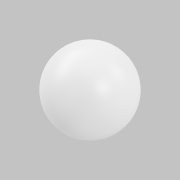
# Autodesk Inventor part: GameDesignFRCBall
Saved by Autodesk Inventor 2021 (Build 250183000, 183)
## iProperties
Created: 2020-01-14
Part Number: GameDesignFRCBall
Material: Generic
Document SubType Name: Modeling
Designer: woodn
Density: 1 g/cm^3
Appearance: Glossy - Gold
Author: woodn
Autodesk Inventor part; units mm, degrees
ref_plane "YZ Plane" through (0, 0, 0) normal (1, 0, 0) x (0, 1, 0)
ref_plane "XZ Plane" through (0, 0, 0) normal (0, 1, 0) x (-1, 0, 0)
ref_plane "XY Plane" through (0, 0, 0) normal (0, 0, 1) x (1, 0, 0)
sketch "Sketch1" plane through (0, 0, 0) normal (1, 0, 0) x (0, 1, 0)
  circle A0 centre (0, 0) radius 50.8
  line L0 (50.8, 0) -> (-50.8, 0)
  dimension "d0" = 101.6
  constraints: 2 end point, 2 point on circle, 1 centre point, 1 coincident, 1 horizontal
  measures "d0" diameter of A0
revolve "Revolution1" add sketch "Sketch1" angle 360 about axis through (0, 50.8, 0) along (0, -1, 0) picked at (9.3339, -25.052) contours A0 L0
body "Solid1"
